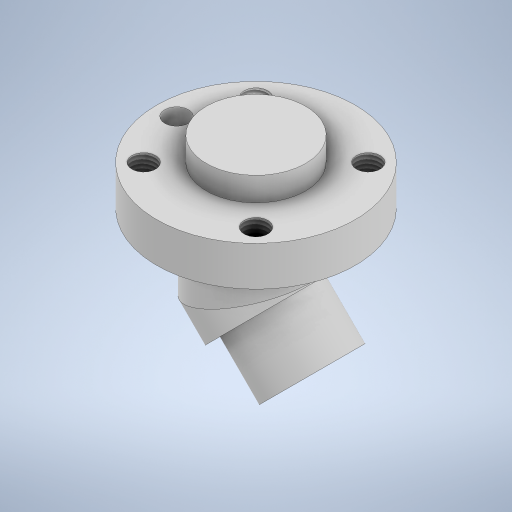
# Autodesk Inventor part: BaseH
Saved by Autodesk Inventor 2024 (Build 280153000, 153)
## iProperties
Created: 2024-02-19
Part Number: BaseH
Material: Genérico
Document SubType Name: Modeling
Designer: Juan David
Density: 1 g/cm^3
Appearance: Valor por defecto
Author: Juan David
Autodesk Inventor part; units mm, degrees
ref_plane "YZ Plane" through (0, 0, 0) normal (1, 0, 0) x (0, 1, 0)
ref_plane "XZ Plane" through (0, 0, 0) normal (0, 1, 0) x (-1, 0, 0)
ref_plane "XY Plane" through (0, 0, 0) normal (0, 0, 1) x (1, 0, 0)
sketch "Boceto1" plane through (0, 0, 0) normal (0, 1, 0) x (-1, 0, 0)
  circle A0 centre (0, 0) radius 25
  circle A1 centre (0, 0) radius 20
  line L0 (0, 0) -> (25, 0)
  line L1 (0, 0) -> (17.6777, -17.6777)
  line L2 (0, 0) -> (25, 0) construction
  line L3 (0, 0) -> (17.6777, 17.6777)
  line L4 (0, 0) -> (25, 0) construction
  line L5 (0, 0) -> (-17.6777, -17.6777)
  line L6 (0, 0) -> (-17.6777, 17.6777)
  circle A2 centre (20, 0) radius 3
  circle A3 centre (14.1421, -14.1421) radius 3
  circle A4 centre (14.1421, 14.1421) radius 3
  circle A5 centre (-14.1421, 14.1421) radius 3
  circle A6 centre (-14.1421, -14.1421) radius 3
  point P0 (16.0984, 11.8677)
  point P1 (11.8677, 16.0984)
  dimension "d0" = 50
  dimension "d1" = 40
  dimension "d2" = 45
  dimension "d3" = 45
  dimension "d4" = 6
  dimension "d5" = 6
  dimension "d6" = 6
  dimension "d7" = 6
  dimension "d8" = 6
  constraints: 14 end point, 10 point on circle, 7 centre point, 7 point on line, 3 horizontal, 2 coincident, 2 equal length
  measures "d0" diameter of A0
  measures "d1" diameter of A1
  measures "d2" angle of L1 L2
  measures "d3" angle of L4 L3
  measures "d4" diameter of A2
  measures "d5" diameter of A3
  measures "d6" diameter of A4
  measures "d7" diameter of A5
  measures "d8" diameter of A6
extrude "Extrusión1" add sketch "Boceto1" along normal blind 10 contours L0 A2 A1 A4 L3 A0 | A0 L1 A3 A1 A2 L0 | L3 A4 A1 A5 L6 A0 | A0 L5 A6 A1 A3 L1 | L6 A5 A1 A6 L5 A0 | A2 L0 L3 A4 A1 | A1 A3 L1 L0 A2 | A4 L3 L6 A5 A1 | A1 A6 L5 L1 A3 | A5 L6 L5 A6 A1
thread "Rosca1"
thread "Rosca2"
thread "Rosca3"
thread "Rosca4"
sketch "Boceto3" plane through (0, 10, 0) normal (0, 1, 0) x (1, 0, 0)
  circle A0 centre (0, 0) radius 12.5
  dimension "d22" = 25
  constraints: 1 centre point, 1 coincident
  measures "d22" diameter of A0
extrude "Extrusión3" add sketch "Boceto3" along normal blind 6
sketch "Boceto7" plane through (0, 0, 0) normal (0, 0, 1) x (1, 0, 0)
  line L0 (0, 0) -> (0, -15)
  line L1 (0, -15) -> (14.1421, -29.1421)
  dimension "d31" = 15
  dimension "d32" = 20
  dimension "d33" = 135
  constraints: 4 end point, 1 vertical
  measures "d31" distance of L0.start L0.end
  measures "d32" distance of L0.end L1.end
  measures "d33" angle of L1 L0
sketch "Boceto8" plane through (0, 0, 0) normal (0, -1, 0) x (1, 0, 0)
  circle A0 centre (0, 0) radius 13.9045
  dimension "d34" = 27.809
  constraints: 1 centre point, 1 coincident
  measures "d34" diameter of A0
sweep "Barrido1" add profiles "Boceto8" path "Boceto7"
sketch "Boceto10" plane through (14.1421, -29.1421, 0) normal (0.7071, -0.7071, 0) x (-0.7071, -0.7071, 0)
  ellipse E0 centre (-17.6777, 0) end of major axis (-17.6777, -25) minor radius 17.6777 projected
  circle A0 centre (0, 0) radius 13.9045
  circle A1 centre (0, 0) radius 10.9045
  point P0 (-10.6066, 0)
  dimension "d40" = 27.809
  dimension "d41" = 21.809
  constraints: 2 centre point, 1 coincident, 1 horizontal alignment, 1 other
  measures "d40" diameter of A0
  measures "d41" diameter of A1
extrude "Extrusión7" cut sketch "Boceto10" against normal blind 14 contours A0 E0 A1 | E0 A1 A0
sketch "Boceto11" plane through (14.1421, -29.1421, 0) normal (0.7071, -0.7071, 0) x (-0.7071, -0.7071, 0)
  ellipse E0 centre (-17.6777, 0) end of major axis (-17.6777, -25) minor radius 17.6777 projected
  circle A0 centre (0, 0) radius 3.05
  point P0 (-10.6066, 0)
  dimension "d44" = 6.1
  constraints: 1 centre point, 1 horizontal alignment, 1 other
  measures "d44" diameter of A0
extrude "Extrusión8" cut sketch "Boceto11" against normal blind 10 contours A0 E0 | E0 A0 picked at (-0.8572, 1.0724) picked at (0.8995, 0.9612)
